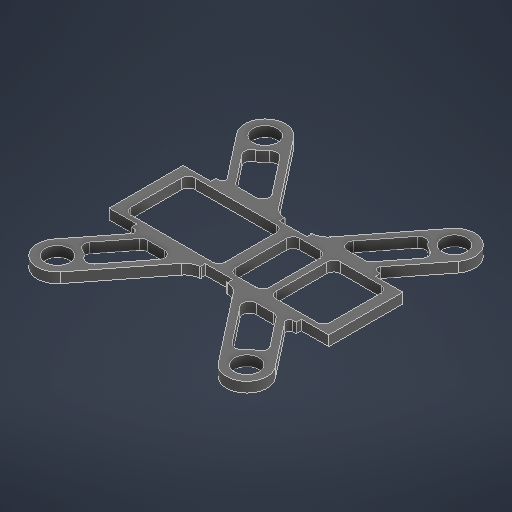
# Autodesk Inventor part: P_DroneCase
Saved by Autodesk Inventor 2026.2 (Build 302298000, 298)
## iProperties
Created: 2025-08-01
Part Number: P_DroneCase
Material: Generisch
Document SubType Name: Modeling
Designer: FAL
Density: 1 g/cm^3
Appearance: Vorgabe
Author: FAL
Autodesk Inventor part; units mm, degrees
ref_plane "YZ Plane" through (0, 0, 0) normal (1, 0, 0) x (0, 1, 0)
ref_plane "XZ Plane" through (0, 0, 0) normal (0, 1, 0) x (-1, 0, 0)
ref_plane "XY Plane" through (0, 0, 0) normal (0, 0, 1) x (1, 0, 0)
sketch "Skizze1" plane through (0, 0, 0) normal (0, 0, 1) x (1, 0, 0)
  line L0 (-32.5, 0) -> (32.5, 0)
  line L1 (32.5, 0) -> (32.5, -12.5)
  line L2 (32.5, -12.5) -> (-32.5, -12.5)
  line L3 (-32.5, -12.5) -> (-32.5, 0)
  line L4 (0, 0) -> (0, -12.5)
  dimension "d0" = 65
  dimension "d1" = 12.5
  constraints: 10 end point, 3 midpoint, 2 parallel, 1 horizontal, 1 perpendicular, 1 point on line
  measures "d0" distance of L1.end L2.end
  measures "d1" distance between parallel lines of L0 L2
extrude "Extrusion1" add sketch "Skizze1" along normal blind 3 contours L0 L1 L2 L4
sketch "Skizze24" plane through (0, 0, 0) normal (0, 0, 1) x (1, 0, 0)
  line L0 (4, 0) -> (28.0108, -30.7324) construction
  line L1 (8.7281, 3.694) -> (32.7389, -27.0385)
  line L2 (23.2827, -34.4264) -> (-0.7281, -3.694)
  arc A0 (8.7281, 3.694) -> (-0.7281, -3.694) centre (4, 0) ccw
  arc A1 (23.2827, -34.4264) -> (32.7389, -27.0385) centre (28.0108, -30.7324) ccw
  line L3 (4, 0) -> (4, -54.7704) construction
  line L4 (32.5, -12.5) -> (32.5, 0) projected
  line L5 (32.5, 0) -> (-37.9025, 0)
  line L6 (0, 0) -> (0, -12.5) projected
  point P0 (16.0054, -15.3662)
  point P1 (11.6141, 0)
  point P2 (-2, 0)
  point P3 (4, 0)
  point P4 (4, -9.7456)
  point P5 (0, -4.6258)
  dimension "d137" = 38
  dimension "d138" = 39
  dimension "d139" = 12
  dimension "d191" = 4
  constraints: 12 end point, 4 point on circle, 4 tangent, 2 centre point, 1 horizontal, 1 horizontal alignment, 1 midpoint, 1 parallel, 1 vertical
  measures "d137" angle of L3 L0
  measures "d138" distance of L0.start L0.end
  measures "d139" distance between parallel lines of L2 L1
  measures "d191" distance between parallel lines of L6 L3
extrude "Extrusion19" add sketch "Skizze24" along normal blind 3 contours L1 A1 L2 L6 L5
sketch "Skizze25" plane through (0, 0, 3) normal (0, 0, 1) x (1, 0, 0)
  arc A0 (23.2827, -34.4264) -> (32.7389, -27.0385) centre (28.0108, -30.7324) ccw projected
  circle A1 centre (28.0108, -30.7324) radius 3.6
  circle A2 centre (28.0108, -30.7324) radius 5.6
  line L0 (22.4459, -30.1067) -> (8.69, -12.5)
  line L1 (0, -12.5) -> (32.5, -12.5) projected
  line L2 (18.8421, -12.5) -> (28.75, -25.1814)
  line L3 (6.152, -12.5) -> (23.2827, -34.4264) projected
  line L4 (32.7389, -27.0385) -> (21.3802, -12.5) projected
  line L5 (9.4713, -13.5) -> (19.6234, -13.5)
  point P0 (0, 0)
  point P1 (-35, -12.5)
  dimension "d142" = 7.2
  dimension "d143" = 2
  dimension "d144" = 2
  dimension "d145" = 2
  dimension "d149" = 1
  constraints: 6 end point, 4 parallel, 4 point on line, 2 centre point, 2 coincident, 2 point on circle
  measures "d142" diameter of A1
  measures "d143" distance between parallel lines of L3 L0
  measures "d144" distance between parallel lines of L4 L2
  measures "d145" radial gap between concentric circles of A1 A2
  measures "d149" distance between parallel lines of L1 L5
extrude "Extrusion20" cut sketch "Skizze25" against normal through all contours L5 L2 A2 L0 | A1
fillet "Rundung14" radius 2 4 edges at (22.4459, -30.1067, 1.5) (28.75, -25.1814, 1.5) (9.4713, -13.5, 1.5) (19.6234, -13.5, 1.5)
sketch "Skizze31" plane through (0, 0, 3) normal (0, 0, 1) x (1, 0, 0)
  line L0 (0, 0) -> (0, -12.5) projected
  line L1 (29.5, 0) -> (0, 0)
  line L2 (0, 0) -> (0, -9.5)
  line L3 (0, -9.5) -> (29.5, -9.5)
  line L4 (29.5, -9.5) -> (29.5, 0)
  line L5 (32.5, -12.5) -> (32.5, 0) projected
  line L6 (0, -12.5) -> (6.152, -12.5) projected
  line L7 (1.5, -9.5) -> (1.5, 0)
  dimension "d186" = 3
  dimension "d187" = 3
  dimension "d195" = 1.5
  constraints: 10 end point, 3 point on line, 2 parallel, 2 perpendicular, 1 horizontal
  measures "d186" distance between parallel lines of L5 L4
  measures "d187" distance between parallel lines of L6 L3
  measures "d195" distance between parallel lines of L0 L7
extrude "Extrusion26" cut sketch "Skizze31" against normal blind 17.5 contours L1 L4 L3 L7
fillet "Rundung24" radius 2 2 edges at (29.5, -9.5, 1.5) (1.5, -9.5, 1.5)
fillet "Rundung25" radius 5 1 edges at (6.152, -12.5, 1.5)
fillet "Rundung26" radius 1 1 edges at (21.3802, -12.5, 1.5)
sketch "Skizze32" plane through (0, 0, 3) normal (0, 0, 1) x (1, 0, 0)
  line L0 (32.5, -12.5) -> (32.5, 0) projected
  line L1 (32.5, -12.5) -> (24.35, -12.5)
  line L2 (24.35, -12.5) -> (24.35, -10.95)
  line L3 (24.35, -10.95) -> (32.5, -10.95)
  line L4 (32.5, -10.95) -> (32.5, -12.5)
  line L5 (0, -12.5) -> (4.1, -12.5)
  line L6 (4.1, -12.5) -> (4.1, -10.95)
  line L7 (4.1, -10.95) -> (0, -10.95)
  line L8 (0, -10.95) -> (0, -12.5)
  point P0 (0, 0)
  dimension "d196" = 1.55
  dimension "d197" = 8.15
  dimension "d200" = 4.1
  constraints: 16 end point, 4 parallel, 2 horizontal, 2 perpendicular, 1 point on line
  measures "d196" distance between parallel lines of L3 L1
  measures "d197" distance between parallel lines of L0 L2
  measures "d200" distance between parallel lines of L8 L6
extrude "Extrusion27" cut sketch "Skizze32" against normal blind 9.25
mirror "Spiegeln5" about plane through (0, 0, 0) normal (1, 0, 0)
sketch "Skizze33" plane through (0, 0, 3) normal (0, 0, 1) x (1, 0, 0)
  line L0 (-27.5, -9.5) -> (-3.5, -9.5) projected
  line L1 (13.5, -9.5) -> (11.5, -9.5)
  line L2 (11.5, -9.5) -> (11.5, 0)
  line L3 (11.5, 0) -> (13.5, 0)
  line L4 (13.5, 0) -> (13.5, -9.5)
  line L5 (-29.5, 0) -> (-29.5, -7.5) projected
  line L6 (1.5, 0) -> (-1.5, 0) projected
  line L7 (29.5, 0) -> (29.5, -7.5) projected
  point P0 (0, 0)
  point P1 (0, 0)
  point P2 (-12, -9.5)
  point P3 (2, 0)
  point P4 (-2, 0)
  dimension "d201" = 2
  dimension "d206" = 16
  constraints: 8 end point, 2 parallel, 2 point on line, 1 horizontal, 1 midpoint, 1 perpendicular
  measures "d201" distance between parallel lines of L4 L2
  measures "d206" distance between parallel lines of L7 L4
extrude "Extrusion28" add sketch "Skizze33" against normal up to surface (3 mm away)
fillet "Rundung28" radius 2 2 edges at (13.5, -9.5, 1.5) (11.5, -9.5, 1.5)
mirror "Spiegeln4" about plane through (0, 0, 0) normal (0, 1, 0)
